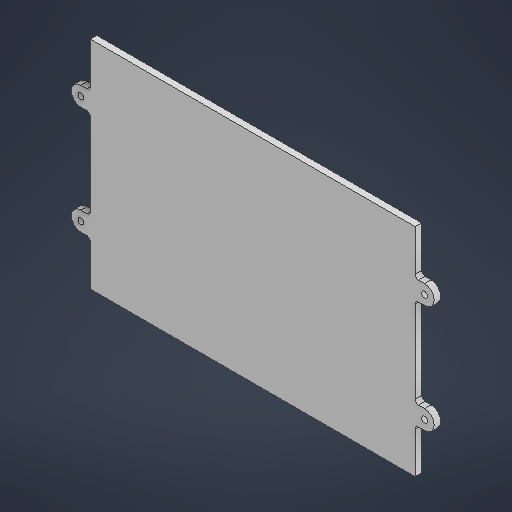
# Autodesk Inventor part: bed-plate
Saved by Autodesk Inventor 2025 (Build 290162000, 162)
## iProperties
Created: 2024-07-18
Part Number: bed-plate
Material: Generic
Document SubType Name: Sheet Metal
Designer: Windows 7 was better
Density: 1 g/cm^3
Appearance: Default
Sheet Metal Rule: Default_mm
Author: Windows 7 was better
Autodesk Inventor part; units mm, degrees
ref_plane "YZ Plane" through (0, 0, 0) normal (1, 0, 0) x (0, 1, 0)
ref_plane "XZ Plane" through (0, 0, 0) normal (0, 1, 0) x (-1, 0, 0)
ref_plane "XY Plane" through (0, 0, 0) normal (0, 0, 1) x (1, 0, 0)
sketch "Sketch1" plane through (0, 0, 0) normal (0, 0, 1) x (1, 0, 0)
  line L0 (150, -100) -> (150, 100)
  line L1 (-150, -100) -> (150, -100)
  line L2 (150, 100) -> (-150, 100)
  line L3 (-150, 100) -> (-150, -100)
  line L4 (0, 100) -> (0, 0) construction
  line L5 (0, 0) -> (0, -100) construction
  line L6 (0, -50) -> (150, -50) construction
  line L7 (0, 50) -> (150, 50) construction
  line L8 (0, 50) -> (-150, 50) construction
  line L9 (0, -50) -> (-150, -50) construction
  line L10 (-150, -50) -> (-158.805, -50) construction
  circle A0 centre (-158.805, -50) radius 8.805
  circle A1 centre (-158.805, -50) radius 2.805
  circle A2 centre (-158.805, 50) radius 2.805
  circle A3 centre (-158.805, 50) radius 8.805
  line L11 (150, -50) -> (158.805, -50) construction
  circle A4 centre (158.805, -50) radius 8.805
  circle A5 centre (158.805, -50) radius 2.805
  circle A6 centre (158.805, 50) radius 8.805
  circle A7 centre (158.805, 50) radius 2.805
  line L12 (158.805, 41.195) -> (150, 41.195)
  line L13 (158.805, 58.805) -> (150, 58.805)
  line L14 (158.805, -41.195) -> (150, -41.195)
  line L15 (158.805, -58.805) -> (150, -58.805)
  line L16 (-158.805, -58.805) -> (-150, -58.805)
  line L17 (-158.805, -41.195) -> (-150, -41.195)
  line L18 (-158.805, 41.195) -> (-150, 41.195)
  line L19 (-158.805, 58.805) -> (-150, 58.805)
  dimension "d0" = 8.805
  dimension "d1" = 5.61
  dimension "d2" = 5.61
  dimension "d3" = 8.805
  dimension "d4" = 5.61
  measures "d0" distance of L9.end L10.end
  measures "d1" diameter of A1
  measures "d2" diameter of A2
  measures "d3" distance of L6.end L11.end
  measures "d4" diameter of A5
extrude "Plate1" add sketch "Sketch1" along normal blind 6
fillet "Corner Round1" radius 3.175 8 edges at (-150, -58.805, 3) (-150, -41.195, 3) (-150, 41.195, 3) (-150, 58.805, 3) (150, 58.805, 3) (150, 41.195, 3) (150, -41.195, 3) (150, -58.805, 3)
equation "\"d7\" = Thickness"
equation "\"BendRadius\" = Thickness"
equation "\"BendReliefWidth\" = Thickness"
equation "\"BendReliefDepth\" = 0.5 * Thickness"
equation "\"CornerReliefSize\" = 4 * Thickness"
equation "\"MinimumRemnant\" = 2 * Thickness"
equation "\"TransitionRadius\" = BendRadius"
equation "\"JacobiRadiusSize\" = BendRadius"
equation "\"GapSize\" = Thickness"
equation "\"Thickness\" = 6"
body "Solid2"
